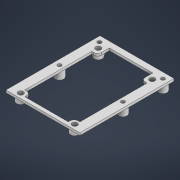
# Autodesk Inventor part: Adapter_PowerManagement
Saved by Autodesk Inventor 2021 (Build 250183000, 183)
## iProperties
Created: 2021-02-21
Part Number: Adapter_PowerManagement
Material: Generisch
Document SubType Name: Modeling
Designer: Ctroi
Density: 1 g/cm^3
Appearance: Vorgabe
Author: Ctroi
Autodesk Inventor part; units mm, degrees
ref_plane "YZ Plane" through (0, 0, 0) normal (1, 0, 0) x (0, 1, 0)
ref_plane "XZ Plane" through (0, 0, 0) normal (0, 1, 0) x (-1, 0, 0)
ref_plane "XY Plane" through (0, 0, 0) normal (0, 0, 1) x (1, 0, 0)
sketch "Skizze1" plane through (0, 0, 0) normal (0, 1, 0) x (-1, 0, 0)
  line L0 (-31.5, 40) -> (31.5, 40)
  line L1 (31.5, 40) -> (31.5, -40)
  line L2 (31.5, -40) -> (-31.5, -40)
  line L3 (-31.5, -40) -> (-31.5, 40)
  line L4 (0, -56) -> (0, 56) projected
  line L5 (-44.1, 0) -> (44.1, 0) projected
  circle A0 centre (27, -35) radius 1.6
  circle A1 centre (-27, -35) radius 1.6
  circle A2 centre (-27, -1) radius 1.6
  circle A3 centre (27, -1) radius 1.6
  point P0 (0, 0)
  dimension "d0" = 63
  dimension "d1" = 80
  dimension "d2" = 3.2
  dimension "d3" = 3.2
  dimension "d4" = 27
  dimension "d5" = 27
  dimension "d6" = 5
  dimension "d7" = 5
  dimension "d8" = 3.2
  dimension "d9" = 3.2
  dimension "d10" = 27
  dimension "d11" = 27
  dimension "d12" = 34
  dimension "d13" = 34
  constraints: 8 end point, 4 centre point, 2 parallel, 1 horizontal, 1 perpendicular, 2 other
  measures "d0" distance of L1.end L2.end
  measures "d1" distance of L0.end L1.end
  measures "d2" diameter of A0
  measures "d3" diameter of A1
  measures "d4" distance from line of L4 A1.centre
  measures "d5" distance from line of L4 A0.centre
  measures "d6" distance from line of L2 A0.centre
  measures "d7" distance from line of L2 A1.centre
  measures "d8" diameter of A2
  measures "d9" diameter of A3
  measures "d10" distance from line of L4 A3.centre
  measures "d11" distance from line of L4 A2.centre
  measures "d12" distance of A1.centre A2.centre
  measures "d13" distance of A0.centre A3.centre
extrude "Extrusion1" add sketch "Skizze1" along normal blind 2 contours L0 L4 L5 A2 L3 | L0 L1 L5 A3 L4 | L5 A2 L4 L2 L3 | L5 A3 L1 L2 L4
sketch "Skizze3" plane through (0, 2, 0) normal (0, 1, 0) x (1, 0, 0)
  circle A0 centre (-23, 30) radius 3.5
  circle A1 centre (23, 30) radius 3.5
  circle A2 centre (23, -36) radius 3.5
  circle A3 centre (-23, -36) radius 3.5
  line L0 (0, 56) -> (0, -56) projected
  line L1 (44.1, 0) -> (-44.1, 0) projected
  line L2 (31.5, 40) -> (-31.5, 40) projected
  point P0 (0, 0)
  dimension "d22" = 7
  dimension "d23" = 7
  dimension "d24" = 7
  dimension "d25" = 7
  dimension "d26" = 23
  dimension "d27" = 23
  dimension "d28" = 23
  dimension "d29" = 23
  dimension "d31" = 10
  dimension "d32" = 10
  dimension "d33" = 66
  dimension "d34" = 66
  constraints: 4 centre point
  measures "d22" diameter of A0
  measures "d23" diameter of A1
  measures "d24" diameter of A2
  measures "d25" diameter of A3
  measures "d26" distance from line of L0 A0.centre
  measures "d27" distance from line of L0 A1.centre
  measures "d28" distance from line of L0 A2.centre
  measures "d29" distance from line of L0 A3.centre
  measures "d31" distance from line of L2 A0.centre
  measures "d32" distance from line of L2 A1.centre
  measures "d33" distance of A0.centre A3.centre
  measures "d34" distance of A1.centre A2.centre
sketch "Skizze2" plane through (0, 0, 0) normal (0, -1, 0) x (1, 0, 0)
  circle A0 centre (27, -1) radius 1.6 projected
  circle A1 centre (27, -35) radius 1.6 projected
  circle A2 centre (-27, -35) radius 1.6 projected
  circle A3 centre (-27, -1) radius 1.6 projected
  circle A4 centre (27, -1) radius 3.5
  circle A5 centre (27, -35) radius 3.5
  circle A6 centre (-27, -1) radius 3.5
  circle A7 centre (-27, -35) radius 3.5
  point P0 (0, 0)
  dimension "d16" = 7
  dimension "d17" = 7
  dimension "d18" = 7
  dimension "d19" = 7
  constraints: 4 centre point, 4 coincident
  measures "d16" diameter of A4
  measures "d17" diameter of A5
  measures "d18" diameter of A6
  measures "d19" diameter of A7
extrude "Extrusion2" add sketch "Skizze2" along normal blind 6.5
extrude "Extrusion3" add sketch "Skizze3" against normal blind 6
sketch "Skizze4" plane through (0, 2, 0) normal (0, 1, 0) x (1, 0, 0)
  arc A0 (23.8957, 33.3835) -> (26.1043, 31.6165) centre (23, 30) ccw projected
  circle A1 centre (23, -36) radius 3.5 projected
  circle A2 centre (-23, -36) radius 3.5 projected
  arc A3 (-26.1043, 31.6165) -> (-23.8957, 33.3835) centre (-23, 30) ccw projected
  circle A4 centre (23, 30) radius 2.25
  circle A5 centre (23, -36) radius 2.25
  circle A6 centre (-23, 30) radius 2.25
  circle A7 centre (-23, -36) radius 2.25
  point P0 (0, 0)
  dimension "d37" = 4.5
  dimension "d38" = 4.5
  dimension "d39" = 4.5
  dimension "d40" = 4.5
  constraints: 4 centre point, 4 coincident
  measures "d37" diameter of A4
  measures "d38" diameter of A5
  measures "d39" diameter of A6
  measures "d40" diameter of A7
extrude "Extrusion4" cut sketch "Skizze4" against normal up to surface (6 mm away) contours A4 | A5 | A6 | A7
sketch "Skizze5" plane through (0, 2, 0) normal (0, 1, 0) x (1, 0, 0)
  line L0 (23.5, -32) -> (23.5, 25)
  line L1 (-23.5, 25) -> (-23.5, -32)
  line L2 (31.5, 40) -> (-31.5, 40) projected
  line L3 (-31.5, -40) -> (31.5, -40) projected
  line L4 (-31.5, 40) -> (-31.5, -40) projected
  line L5 (31.5, -40) -> (31.5, 40) projected
  line L6 (18.5, -32) -> (18.5, -37)
  line L7 (18.5, -37) -> (-18.5, -37)
  line L8 (-18.5, -37) -> (-18.5, -32)
  line L9 (18.5, 25) -> (18.5, 35)
  line L10 (18.5, 35) -> (-18.5, 35)
  line L11 (-18.5, 35) -> (-18.5, 25)
  line L12 (-23.5, -32) -> (-18.5, -32)
  line L13 (18.5, -32) -> (23.5, -32)
  line L14 (23.5, 25) -> (18.5, 25)
  line L15 (-18.5, 25) -> (-23.5, 25)
  point P0 (0, 0)
  dimension "d45" = 8
  dimension "d46" = 8
  dimension "d49" = 3
  dimension "d50" = 13
  dimension "d51" = 13
  dimension "d52" = 13
  dimension "d53" = 13
  dimension "d54" = 5
  dimension "d55" = 8
  dimension "d56" = 8
  dimension "d57" = 15
  dimension "d58" = 15
  constraints: 24 end point, 7 parallel, 2 horizontal, 2 perpendicular
  measures "d45" distance between parallel lines of L4 L1
  measures "d46" distance between parallel lines of L5 L0
  measures "d49" distance between parallel lines of L3 L7
  measures "d50" distance between parallel lines of L4 L8
  measures "d51" distance between parallel lines of L5 L6
  measures "d52" distance between parallel lines of L4 L11
  measures "d53" distance between parallel lines of L5 L9
  measures "d54" distance between parallel lines of L2 L10
  measures "d55" distance between parallel lines of L3 L12
  measures "d56" distance between parallel lines of L3 L13
  measures "d57" distance between parallel lines of L2 L14
  measures "d58" distance between parallel lines of L2 L15
extrude "Extrusion5" cut sketch "Skizze5" against normal up to surface (2 mm away) contours L13 L6 L7 L8 L12 L1 L15 L11 L10 L9 L14 L0
fillet "Rundung1" radius 3.5 4 edges at (18.5, 1, 32) (18.5, 1, -25) (-18.5, 1, -25) (-18.5, 1, 32)
